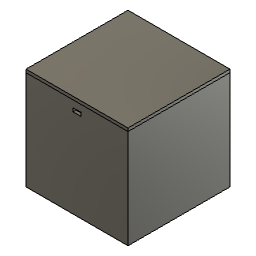
skeleton (Autodesk Fusion 360 design; units mm, degrees)
Autodesk Fusion 360 part; units mm, degrees
sketch "Sketch1" plane through (0, 0, 0) normal (0, 1, 0) x (1, 0, 0)
  line L0 (-50, -50) -> (50, -50)
  line L1 (50, -50) -> (50, 50)
  line L2 (50, 50) -> (-50, 50)
  line L3 (-50, 50) -> (-50, -50)
  line L4 (-50, -50) -> (50, 50) construction
  line L5 (50, -50) -> (-50, 50) construction
  line L6 (-33.25, 0) -> (-50, 0) construction
  line L7 (-41.625, 50) -> (-41.625, 0) construction
  line L8 (-50, 30) -> (-41.625, 30) construction
  line L9 (-50, 10) -> (-41.625, 10) construction
  line L10 (-50, -10) -> (-41.625, -10) construction
  line L11 (-50, -30) -> (-41.625, -30) construction
  line L12 (-44.725, 26.9) -> (-38.525, 26.9)
  line L13 (-38.525, 26.9) -> (-38.525, 33.1)
  line L14 (-38.525, 33.1) -> (-44.725, 33.1)
  line L15 (-44.725, 33.1) -> (-44.725, 26.9)
  line L16 (-44.725, 26.9) -> (-38.525, 33.1) construction
  line L17 (-38.525, 26.9) -> (-44.725, 33.1) construction
  line L18 (-44.725, 6.9) -> (-38.525, 6.9)
  line L19 (-38.525, 6.9) -> (-38.525, 13.1)
  line L20 (-38.525, 13.1) -> (-44.725, 13.1)
  line L21 (-44.725, 13.1) -> (-44.725, 6.9)
  line L22 (-44.725, 6.9) -> (-38.525, 13.1) construction
  line L23 (-38.525, 6.9) -> (-44.725, 13.1) construction
  line L24 (-44.725, -13.1) -> (-38.525, -13.1)
  line L25 (-38.525, -13.1) -> (-38.525, -6.9)
  line L26 (-38.525, -6.9) -> (-44.725, -6.9)
  line L27 (-44.725, -6.9) -> (-44.725, -13.1)
  line L28 (-44.725, -13.1) -> (-38.525, -6.9) construction
  line L29 (-38.525, -13.1) -> (-44.725, -6.9) construction
  line L30 (-43.645, -24.16) -> (-39.605, -24.16)
  line L31 (-39.605, -24.16) -> (-39.605, -35.84)
  line L32 (-39.605, -35.84) -> (-43.645, -35.84)
  line L33 (-43.645, -35.84) -> (-43.645, -24.16)
  line L34 (-43.645, -24.16) -> (-39.605, -35.84) construction
  line L35 (-39.605, -24.16) -> (-43.645, -35.84) construction
  line L36 (-47, -47) -> (47, -47)
  line L37 (47, -47) -> (47, 47)
  line L38 (47, 47) -> (-47, 47)
  line L39 (-47, 47) -> (-47, -47)
  line L40 (0, 0) -> (-32.9655, 4.34) construction
  line L41 (-25.8747, -2.5491) -> (-33.0657, -3.4958)
  line L42 (-25.6528, -4.2346) -> (-32.8438, -5.1813)
  line L43 (-29.4702, -3.0225) -> (-29.2483, -4.708) construction
  line L44 (-23.6827, -10.7297) -> (-30.3837, -13.5054)
  line L45 (-24.3333, -9.1592) -> (-31.0342, -11.9348)
  line L46 (-20.0987, -16.4937) -> (-25.8529, -20.9091)
  line L47 (-21.1336, -15.145) -> (-26.8878, -19.5604)
  line L48 (-15.145, -21.1336) -> (-19.5604, -26.8878)
  line L49 (-16.4937, -20.0987) -> (-20.9091, -25.8529)
  line L50 (-9.1592, -24.3333) -> (-11.9348, -31.0342)
  line L51 (-10.7297, -23.6827) -> (-13.5054, -30.3837)
  line L52 (-2.5491, -25.8747) -> (-3.4958, -33.0657)
  line L53 (-4.2346, -25.6528) -> (-5.1813, -32.8438)
  line L54 (4.2346, -25.6528) -> (5.1813, -32.8438)
  line L55 (2.5491, -25.8747) -> (3.4958, -33.0657)
  line L56 (10.7297, -23.6827) -> (13.5054, -30.3837)
  line L57 (9.1592, -24.3333) -> (11.9348, -31.0342)
  line L58 (16.4937, -20.0987) -> (20.9091, -25.8529)
  line L59 (15.145, -21.1336) -> (19.5604, -26.8878)
  line L60 (21.1336, -15.145) -> (26.8878, -19.5604)
  line L61 (20.0987, -16.4937) -> (25.8529, -20.9091)
  line L62 (24.3333, -9.1592) -> (31.0342, -11.9348)
  line L63 (23.6827, -10.7297) -> (30.3837, -13.5054)
  line L64 (25.8747, -2.5491) -> (33.0657, -3.4958)
  line L65 (25.6528, -4.2346) -> (32.8438, -5.1813)
  line L66 (25.6528, 4.2346) -> (32.8438, 5.1813)
  line L67 (25.8747, 2.5491) -> (33.0657, 3.4958)
  line L68 (23.6827, 10.7297) -> (30.3837, 13.5054)
  line L69 (24.3333, 9.1592) -> (31.0342, 11.9348)
  line L70 (20.0987, 16.4937) -> (25.8529, 20.9091)
  line L71 (21.1336, 15.145) -> (26.8878, 19.5604)
  line L72 (15.145, 21.1336) -> (19.5604, 26.8878)
  line L73 (16.4937, 20.0987) -> (20.9091, 25.8529)
  line L74 (9.1592, 24.3333) -> (11.9348, 31.0342)
  line L75 (10.7297, 23.6827) -> (13.5054, 30.3837)
  line L76 (2.5491, 25.8747) -> (3.4958, 33.0657)
  line L77 (4.2346, 25.6528) -> (5.1813, 32.8438)
  line L78 (-4.2346, 25.6528) -> (-5.1813, 32.8438)
  line L79 (-2.5491, 25.8747) -> (-3.4958, 33.0657)
  line L80 (-10.7297, 23.6827) -> (-13.5054, 30.3837)
  line L81 (-9.1592, 24.3333) -> (-11.9348, 31.0342)
  line L82 (-16.4937, 20.0987) -> (-20.9091, 25.8529)
  line L83 (-15.145, 21.1336) -> (-19.5604, 26.8878)
  line L84 (-21.1336, 15.145) -> (-26.8878, 19.5604)
  line L85 (-20.0987, 16.4937) -> (-25.8529, 20.9091)
  line L86 (-24.3333, 9.1592) -> (-31.0342, 11.9348)
  line L87 (-23.6827, 10.7297) -> (-30.3837, 13.5054)
  line L88 (-25.8747, 2.5491) -> (-33.0657, 3.4958)
  line L89 (-25.6528, 4.2346) -> (-32.8438, 5.1813)
  line L90 (0, 0) -> (-25.7776, -3.3937) construction
  line L91 (-29.3593, -3.8652) -> (-32.9655, -4.34) construction
  arc A0 (-25.6528, -4.2346) -> (-24.3333, -9.1592) centre (0, 0) ccw
  arc A1 (-32.8438, -5.1813) -> (-31.0342, -11.9348) centre (0, 0) ccw
  arc A2 (-30.3837, -13.5054) -> (-26.8878, -19.5604) centre (0, 0) ccw
  arc A3 (-23.6827, -10.7297) -> (-21.1336, -15.145) centre (0, 0) ccw
  arc A4 (-20.0987, -16.4937) -> (-16.4937, -20.0987) centre (0, 0) ccw
  arc A5 (-25.8529, -20.9091) -> (-20.9091, -25.8529) centre (0, 0) ccw
  arc A6 (-15.145, -21.1336) -> (-10.7297, -23.6827) centre (0, 0) ccw
  arc A7 (-19.5604, -26.8878) -> (-13.5054, -30.3837) centre (0, 0) ccw
  arc A8 (-11.9348, -31.0342) -> (-5.1813, -32.8438) centre (0, 0) ccw
  arc A9 (-9.1592, -24.3333) -> (-4.2346, -25.6528) centre (0, 0) ccw
  arc A10 (-2.5491, -25.8747) -> (2.5491, -25.8747) centre (0, 0) ccw
  arc A11 (-3.4958, -33.0657) -> (3.4958, -33.0657) centre (0, 0) ccw
  arc A12 (5.1813, -32.8438) -> (11.9348, -31.0342) centre (0, 0) ccw
  arc A13 (4.2346, -25.6528) -> (9.1592, -24.3333) centre (0, 0) ccw
  arc A14 (10.7297, -23.6827) -> (15.145, -21.1336) centre (0, 0) ccw
  arc A15 (13.5054, -30.3837) -> (19.5604, -26.8878) centre (0, 0) ccw
  arc A16 (20.9091, -25.8529) -> (25.8529, -20.9091) centre (0, 0) ccw
  arc A17 (16.4937, -20.0987) -> (20.0987, -16.4937) centre (0, 0) ccw
  arc A18 (21.1336, -15.145) -> (23.6827, -10.7297) centre (0, 0) ccw
  arc A19 (26.8878, -19.5604) -> (30.3837, -13.5054) centre (0, 0) ccw
  arc A20 (31.0342, -11.9348) -> (32.8438, -5.1813) centre (0, 0) ccw
  arc A21 (24.3333, -9.1592) -> (25.6528, -4.2346) centre (0, 0) ccw
  arc A22 (25.8747, -2.5491) -> (25.8747, 2.5491) centre (0, 0) ccw
  arc A23 (33.0657, -3.4958) -> (33.0657, 3.4958) centre (0, 0) ccw
  arc A24 (32.8438, 5.1813) -> (31.0342, 11.9348) centre (0, 0) ccw
  arc A25 (25.6528, 4.2346) -> (24.3333, 9.1592) centre (0, 0) ccw
  arc A26 (23.6827, 10.7297) -> (21.1336, 15.145) centre (0, 0) ccw
  arc A27 (30.3837, 13.5054) -> (26.8878, 19.5604) centre (0, 0) ccw
  arc A28 (25.8529, 20.9091) -> (20.9091, 25.8529) centre (0, 0) ccw
  arc A29 (20.0987, 16.4937) -> (16.4937, 20.0987) centre (0, 0) ccw
  arc A30 (15.145, 21.1336) -> (10.7297, 23.6827) centre (0, 0) ccw
  arc A31 (19.5604, 26.8878) -> (13.5054, 30.3837) centre (0, 0) ccw
  arc A32 (9.1592, 24.3333) -> (4.2346, 25.6528) centre (0, 0) ccw
  arc A33 (11.9348, 31.0342) -> (5.1813, 32.8438) centre (0, 0) ccw
  arc A34 (2.5491, 25.8747) -> (-2.5491, 25.8747) centre (0, 0) ccw
  arc A35 (3.4958, 33.0657) -> (-3.4958, 33.0657) centre (0, 0) ccw
  arc A36 (-4.2346, 25.6528) -> (-9.1592, 24.3333) centre (0, 0) ccw
  arc A37 (-5.1813, 32.8438) -> (-11.9348, 31.0342) centre (0, 0) ccw
  arc A38 (-13.5054, 30.3837) -> (-19.5604, 26.8878) centre (0, 0) ccw
  arc A39 (-10.7297, 23.6827) -> (-15.145, 21.1336) centre (0, 0) ccw
  arc A40 (-16.4937, 20.0987) -> (-20.0987, 16.4937) centre (0, 0) ccw
  arc A41 (-20.9091, 25.8529) -> (-25.8529, 20.9091) centre (0, 0) ccw
  arc A42 (-26.8878, 19.5604) -> (-30.3837, 13.5054) centre (0, 0) ccw
  arc A43 (-21.1336, 15.145) -> (-23.6827, 10.7297) centre (0, 0) ccw
  arc A44 (-31.0342, 11.9348) -> (-32.8438, 5.1813) centre (0, 0) ccw
  arc A45 (-33.0657, 3.4958) -> (-33.0657, -3.4958) centre (0, 0) ccw
  arc A46 (-24.3333, 9.1592) -> (-25.6528, 4.2346) centre (0, 0) ccw
  arc A47 (-25.8747, 2.5491) -> (-25.8747, -2.5491) centre (0, 0) ccw
  point P0 (-41.625, 30)
  point P1 (-41.625, 10)
  point P2 (-41.625, -10)
  point P3 (-41.625, -30)
  dimension "d3" = 66.5
  dimension "d4" = 52
  dimension "d5" = 100
  dimension "d6" = 100
  dimension "d7" = 20
  dimension "d10" = 0
  dimension "d11" = -20
  dimension "d12" = 6.2
  dimension "d13" = 6.2
  dimension "d14" = 6.2
  dimension "d15" = 6.2
  dimension "d16" = 6.2
  dimension "d17" = 6.2
  dimension "d18" = 4.04
  dimension "d19" = 11.68
  dimension "d20" = -3
  dimension "d21" = 15
  dimension "d22" = 7.5
  dimension "d23" = 1.7
  dimension "d24" = 0.85
  dimension "d26" = 360
  constraint coincident L40.start L90.start
  constraint concentric A0 A1
  constraint horizontal L0
  constraint perpendicular L0 L1
  constraint parallel L0 L2
  constraint parallel L1 L3
  constraint coincident L4 L40.start
  constraint coincident L5 L40.start
  constraint coincident L6.start A1
  constraint midpoint L3 L6.end
  constraint horizontal L6
  constraint coincident L2 L7.start
  constraint midpoint L6 L7.end
  constraint vertical L7
  constraint coincident L3 L8.start
  constraint coincident L7 P0
  constraint perpendicular L7 L8
  constraint horizontal L12
  constraint perpendicular L12 L13
  constraint parallel L12 L14
  constraint parallel L13 L15
  constraint coincident L16 P0
  constraint coincident L17 P0
  constraint coincident P0 L8.end
  constraint horizontal L18
  constraint perpendicular L18 L19
  constraint parallel L18 L20
  constraint parallel L19 L21
  constraint coincident L22 P1
  constraint coincident L23 P1
  constraint coincident P1 L9.end
  constraint horizontal L24
  constraint perpendicular L24 L25
  constraint parallel L24 L26
  constraint parallel L25 L27
  constraint coincident L28 P2
  constraint coincident L29 P2
  constraint coincident P2 L10.end
  constraint horizontal L30
  constraint perpendicular L30 L31
  constraint parallel L30 L32
  constraint parallel L31 L33
  constraint coincident L34 P3
  constraint coincident L35 P3
  constraint coincident P3 L11.end
  constraint coincident L40.end A1
  constraint parallel L41 L90
  constraint parallel L42 L90
  constraint midpoint L41 L43.start
  constraint midpoint L42 L43.end
  constraint coincident L43 L91.start
  constraint collinear L90 L91
  constraint concentric A0 A3
  constraint concentric A1 A2
  constraint concentric A2 A5
  constraint concentric A3 A4
  constraint concentric A4 A6
  constraint concentric A5 A7
  constraint concentric A6 A9
  constraint concentric A7 A8
  constraint concentric A8 A11
  constraint concentric A9 A10
  constraint concentric A10 A13
  constraint concentric A11 A12
  constraint concentric A12 A15
  constraint concentric A13 A14
  constraint concentric A14 A17
  constraint concentric A15 A16
  constraint concentric A16 A19
  constraint concentric A17 A18
  constraint concentric A18 A21
  constraint concentric A19 A20
  constraint concentric A20 A23
  constraint concentric A21 A22
  constraint concentric A22 A25
  constraint concentric A23 A24
  constraint concentric A24 A27
  constraint concentric A25 A26
  constraint concentric A26 A29
  constraint concentric A27 A28
  constraint concentric A28 A31
  constraint concentric A29 A30
  constraint concentric A30 A32
  constraint concentric A31 A33
  constraint concentric A32 A34
  constraint concentric A33 A35
  constraint concentric A34 A36
  constraint concentric A35 A37
  constraint concentric A36 A39
  constraint concentric A37 A38
  constraint concentric A38 A41
  constraint concentric A39 A40
  constraint concentric A40 A43
  constraint concentric A41 A42
  constraint concentric A42 A44
  constraint concentric A43 A46
  constraint concentric A44 A45
  constraint concentric A46 A47
  measures "d3" diameter of A1
  measures "d4" diameter of A0
  measures "d5" distance of L1.end L2.end
  measures "d6" distance of L0.end L1.end
  measures "d7" distance of L2 L8
  measures "d12" distance of L13.end L14.end
  measures "d13" distance of L12.end L13.end
  measures "d14" distance of L19.end L20.end
  measures "d15" distance of L18.end L19.end
  measures "d16" distance of L25.end L26.end
  measures "d17" distance of L24.end L25.end
  measures "d18" distance of L31.end L32.end
  measures "d19" distance of L30.end L31.end
  measures "d21" angle of L40 L90
  measures "d22" angle of L6 L90
  measures "d23" distance of L41 L42
  measures "d24" distance of L42 L90
extrude "Extrude1" add sketch "Sketch1" along normal blind 3 contours L36 L37 L38 L39 makes body 1
extrude "Extrude2" add sketch "Sketch1" along normal blind 97 contours L0 L1 L2 L3 bodies 1
sketch "Sketch2" plane through (0, 97, 0) normal (0, 1, 0) x (-1, 0, 0)
  line L0 (47, 47) -> (47, -47)
  line L1 (47, -47) -> (-47, -47)
  line L2 (-47, -47) -> (-47, 47)
  line L3 (-47, 47) -> (47, 47)
  line L4 (50, -50) -> (50, 50)
  line L5 (50, 50) -> (-50, 50)
  line L6 (-50, 50) -> (-50, -50)
  line L7 (-50, -50) -> (50, -50)
  line L8 (-50, 50) -> (-50, -50)
  line L9 (50, 50) -> (-50, 50)
  line L10 (50, -50) -> (50, 50)
  line L11 (-50, -50) -> (50, -50)
extrude "Extrude3" add sketch "Sketch2" along normal blind 3 separate body contours L0 L1 L2 L3 | L4 L5 L6 L7 L8 L9 L10 L11 makes body 2
sketch "Sketch3" plane through (0, 97, 0) normal (0, -1, 0) x (1, 0, 0)
  line L0 (-50, -50) -> (50, -50)
  line L1 (50, -50) -> (50, 50)
  line L2 (50, 50) -> (-50, 50)
  line L3 (-50, 50) -> (-50, -50)
  line L4 (47, -47) -> (47, 47)
  line L5 (47, 47) -> (-47, 47)
  line L6 (-47, 47) -> (-47, -47)
  line L7 (-47, -47) -> (47, -47)
  line L8 (0, -47) -> (0, 47) construction
  line L9 (3.75, -46.8) -> (-3.75, -46.8)
  line L10 (-3.75, -46.8) -> (-3.75, -43.8)
  line L11 (-3.75, -43.8) -> (3.75, -43.8)
  line L12 (3.75, -43.8) -> (3.75, -46.8)
  line L13 (47, 0) -> (-47, 0) construction
  line L14 (-3.75, 43.8) -> (3.75, 43.8)
  line L15 (-3.75, 46.8) -> (-3.75, 43.8)
  line L16 (3.75, 46.8) -> (-3.75, 46.8)
  line L17 (3.75, 43.8) -> (3.75, 46.8)
  dimension "d33" = 0.2
  dimension "d34" = 7.5
  dimension "d35" = 3.75
  dimension "d36" = 3
  constraint midpoint L7 L8.start
  constraint midpoint L5 L8.end
  constraint horizontal L9
  constraint vertical L10
  constraint horizontal L11
  constraint vertical L12
  constraint midpoint L4 L13.start
  constraint midpoint L6 L13.end
  constraint symmetric L9.start L13 L16.start
  constraint symmetric L9.end L13 L15.start
  constraint symmetric L10.end L13 L14.start
  constraint symmetric L11.end L13 L14.end
  measures "d33" distance of L7 L9
  measures "d34" distance of L10 L12
  measures "d35" distance of L8 L10
  measures "d36" distance of L9.end L10.end
extrude "Extrude4" add sketch "Sketch3" along normal blind 10 contours L9 L10 L11 L12 | L14 L15 L16 L17 bodies 2
sketch "Sketch4" plane through (3.75, 0, 0) normal (1, 0, 0) x (0, 0, -1)
  line L0 (46.8, 97) -> (43.8, 97)
  line L1 (43.8, 97) -> (43.8, 87)
  line L2 (43.8, 87) -> (46.8, 87)
  line L3 (46.8, 87) -> (46.8, 97)
  line L4 (46.8, 90) -> (48.55, 90)
  line L5 (48.55, 90) -> (46.8, 87)
  line L6 (-43.8, 97) -> (-46.8, 97)
  line L7 (-46.8, 97) -> (-46.8, 87)
  line L8 (-46.8, 87) -> (-43.8, 87)
  line L9 (-43.8, 87) -> (-43.8, 97)
  line L10 (43.8, 87) -> (-43.8, 87) construction
  line L11 (0, 87) -> (0, 80) construction
  line L12 (-48.55, 90) -> (-46.8, 87)
  line L13 (-46.8, 90) -> (-48.55, 90)
  dimension "d39" = 1.75
  dimension "d40" = 3
  constraint coincident L3 L4.start
  constraint perpendicular L3 L4
  constraint coincident L2.end L3.start
  constraint coincident L1.end L2.start
  constraint coincident L8.end L9.start
  constraint midpoint L10 L11.start
  constraint perpendicular L10 L11
  constraint symmetric L4.start L11 L13.start
  constraint symmetric L4.end L11 L12.start
  constraint symmetric L2.end L11 L7.end
  measures "d39" distance of L4.start L4.end
  measures "d40" vertical distance of L4.end L2.end
extrude "Extrude5" add sketch "Sketch4" against normal blind 7.5 contours L3 L4 L5 | L7 L12 L13 bodies 2
sketch "Sketch5" plane through (0, 0, -50) normal (0, 0, -1) x (-1, 0, 0)
  line L0 (-50, 0) -> (50, 0)
  line L1 (50, 0) -> (50, 97)
  line L2 (50, 97) -> (-50, 97)
  line L3 (-50, 97) -> (-50, 0)
  line L4 (-3.75, 90) -> (-3.75, 87)
  line L5 (-3.75, 87) -> (3.75, 87)
  line L6 (3.75, 87) -> (3.75, 90)
  line L7 (3.75, 90) -> (-3.75, 90)
  line L8 (4, 86.75) -> (4, 90.25)
  line L9 (4, 90.25) -> (-4, 90.25)
  line L10 (-4, 90.25) -> (-4, 86.75)
  line L11 (-4, 86.75) -> (4, 86.75)
  dimension "d43" = 0.25
extrude "Extrude6" cut sketch "Sketch5" against normal blind 180 contours L4 L5 L6 L7 | L8 L9 L10 L11 bodies 1
equation "d24 = ( 1.7 / 2 ) * 1 mm"
equation "d35 = ( 7.5 / 2 ) * 1 mm"
